Autodesk Inventor part; units mm, degrees
(part 3 of 5)
  line L1755 (-94.2698, 37.7318) -> (-93.9009, 37.14)
  line L1756 (-93.9009, 37.14) -> (-93.3437, 36.7396)
  line L1757 (-93.3437, 36.7396) -> (-92.5984, 36.5308)
  line L1758 (-92.5984, 36.5308) -> (-92.3338, 35.8693)
  line L1759 (-92.3338, 35.8693) -> (-93.5244, 33.2235)
  line L1760 (-93.5244, 33.2235) -> (-94.7873, 31.4902)
  line L1761 (-94.7873, 31.4902) -> (-95.5088, 29.5193)
  line L1762 (-95.5088, 29.5193) -> (-94.1859, 29.387)
  line L1763 (-94.1859, 29.387) -> (-93.4865, 28.8762)
  line L1764 (-93.4865, 28.8762) -> (-92.8566, 28.7721)
  line L1765 (-92.8566, 28.7721) -> (-92.2959, 29.0747)
  line L1766 (-92.2959, 29.0747) -> (-91.8046, 29.7839)
  line L1767 (-91.8046, 29.7839) -> (-92.3407, 30.6542)
  line L1768 (-92.3407, 30.6542) -> (-92.5855, 31.5617)
  line L1769 (-92.5855, 31.5617) -> (-92.5391, 32.5063)
  line L1770 (-92.5391, 32.5063) -> (-92.2015, 33.4881)
  line L1771 (-92.2015, 33.4881) -> (-91.5401, 33.7526)
  line L1772 (-91.5401, 33.7526) -> (-90.8786, 33.4881)
  line L1773 (-90.8786, 33.4881) -> (-90.2171, 30.0485)
  line L1774 (-90.2171, 30.0485) -> (-89.2902, 29.4549)
  line L1775 (-89.2902, 29.4549) -> (-88.6296, 28.5933)
  line L1776 (-88.6296, 28.5933) -> (-89.4059, 27.4096)
  line L1777 (-89.4059, 27.4096) -> (-90.3494, 26.3443)
  line L1778 (-90.3494, 26.3443) -> (-90.2708, 24.8832)
  line L1779 (-90.2708, 24.8832) -> (-90.399, 23.448)
  line L1780 (-90.399, 23.448) -> (-90.7339, 22.0389)
  line L1781 (-90.7339, 22.0389) -> (-91.2755, 20.6558)
  line L1782 (-91.2755, 20.6558) -> (-90.4507, 18.0829)
  line L1783 (-90.4507, 18.0829) -> (-89.1588, 15.761)
  line L1784 (-89.1588, 15.761) -> (-91.2755, 9.2787)
  line L1785 (-91.2755, 9.2787) -> (-91.0109, 8.6173)
  line L1786 (-91.0109, 8.6173) -> (-91.4592, 5.8191)
  line L1787 (-91.4592, 5.8191) -> (-92.0692, 3.061)
  line L1788 (-92.0692, 3.061) -> (-91.2286, 3.2382)
  line L1789 (-91.2286, 3.2382) -> (-90.614, 3.8548)
  line L1790 (-90.614, 3.8548) -> (-90.0294, 5.553)
  line L1791 (-90.0294, 5.553) -> (-89.0265, 7.0298)
  line L1792 (-89.0265, 7.0298) -> (-88.0062, 10.279)
  line L1793 (-88.0062, 10.279) -> (-87.439, 13.6444)
  line L1794 (-87.439, 13.6444) -> (-87.0421, 13.9089)
  line L1795 (-87.0421, 13.9089) -> (-86.9263, 10.5984)
  line L1796 (-86.9263, 10.5984) -> (-87.3067, 7.2944)
  line L1797 (-87.3067, 7.2944) -> (-87.1071, 5.8402)
  line L1798 (-87.1071, 5.8402) -> (-86.513, 4.5162)
  line L1799 (-86.513, 4.5162) -> (-87.5068, 1.3222)
  line L1800 (-87.5068, 1.3222) -> (-88.1005, -1.966)
  line L1801 (-29.0985, 51.4797) -> (-28.5184, 51.322)
  line L1802 (-28.5184, 51.322) -> (-28.0401, 50.9506)
  line L1803 (-28.0401, 50.9506) -> (-26.865, 49.3772)
  line L1804 (-26.865, 49.3772) -> (-25.9235, 47.6433)
  line L1805 (-25.9235, 47.6433) -> (-26.2095, 47.3714)
  line L1806 (-26.2095, 47.3714) -> (-26.5849, 47.2464)
  line L1807 (-26.5849, 47.2464) -> (-27.696, 47.8294)
  line L1808 (-27.696, 47.8294) -> (-28.7016, 48.5693)
  line L1809 (-28.7016, 48.5693) -> (-29.1503, 48.3856)
  line L1810 (-29.1503, 48.3856) -> (-29.4953, 48.0401)
  line L1811 (-29.4953, 48.0401) -> (-30.4738, 46.006)
  line L1812 (-30.4738, 46.006) -> (-31.612, 44.0714)
  line L1813 (-31.612, 44.0714) -> (-31.7443, 41.161)
  line L1814 (-31.7443, 41.161) -> (-32.8973, 41.4727)
  line L1815 (-32.8973, 41.4727) -> (-33.9933, 41.9547)
  line L1816 (-33.9933, 41.9547) -> (-34.3693, 45.4109)
  line L1817 (-34.3693, 45.4109) -> (-34.9193, 48.8339)
  line L1818 (-34.9193, 48.8339) -> (-34.6686, 49.4453)
  line L1819 (-34.6686, 49.4453) -> (-34.2984, 49.7814)
  line L1820 (-34.2984, 49.7814) -> (-33.8087, 49.8422)
  line L1821 (-33.8087, 49.8422) -> (-33.1995, 49.6276)
  line L1822 (-33.1995, 49.6276) -> (-32.2735, 45.9235)
  line L1823 (-32.2735, 45.9235) -> (-31.5452, 46.3563)
  line L1824 (-31.5452, 46.3563) -> (-31.1041, 46.9415)
  line L1825 (-31.1041, 46.9415) -> (-30.9499, 47.6792)
  line L1826 (-30.9499, 47.6792) -> (-31.0828, 48.5693)
  line L1827 (-31.0828, 48.5693) -> (-31.3153, 49.1092)
  line L1828 (-31.3153, 49.1092) -> (-31.3486, 49.6419)
  line L1829 (-31.3486, 49.6419) -> (-31.1829, 50.1675)
  line L1830 (-31.1829, 50.1675) -> (-30.8183, 50.686)
  line L1831 (-30.8183, 50.686) -> (-29.0985, 51.4797)
  line L1832 (-128.8463, 51.2151) -> (-125.6713, 51.2151)
  line L1833 (-125.6713, 51.2151) -> (-125.6713, 50.4214)
  line L1834 (-125.6713, 50.4214) -> (-128.5817, 50.2891)
  line L1835 (-128.5817, 50.2891) -> (-128.8138, 50.7213)
  line L1836 (-128.8138, 50.7213) -> (-128.8463, 51.2151)
  line L1837 (2.9161, 49.6276) -> (4.254, 49.6112)
  line L1838 (4.254, 49.6112) -> (5.5619, 49.3631)
  line L1839 (5.5619, 49.3631) -> (5.7224, 48.3373)
  line L1840 (5.7224, 48.3373) -> (5.6437, 47.356)
  line L1841 (5.6437, 47.356) -> (5.3256, 46.4191)
  line L1842 (5.3256, 46.4191) -> (4.7682, 45.5266)
  line L1843 (4.7682, 45.5266) -> (4.3713, 45.3942)
  line L1844 (4.3713, 45.3942) -> (3.9744, 45.5266)
  line L1845 (3.9744, 45.5266) -> (2.3869, 48.3047)
  line L1846 (2.3869, 48.3047) -> (2.9161, 49.6276)
  line L1847 (-138.1067, 49.3631) -> (-136.9146, 49.1321)
  line L1848 (-136.9146, 49.1321) -> (-135.8577, 48.5693)
  line L1849 (-135.8577, 48.5693) -> (-135.3932, 47.0503)
  line L1850 (-135.3932, 47.0503) -> (-135.3486, 45.5738)
  line L1851 (-135.3486, 45.5738) -> (-135.7239, 44.1398)
  line L1852 (-135.7239, 44.1398) -> (-136.5192, 42.7485)
  line L1853 (-136.5192, 42.7485) -> (-136.8754, 42.4036)
  line L1854 (-136.8754, 42.4036) -> (-137.2587, 42.2446)
  line L1855 (-137.2587, 42.2446) -> (-137.6691, 42.2714)
  line L1856 (-137.6691, 42.2714) -> (-138.1067, 42.4839)
  line L1857 (-138.1067, 42.4839) -> (-138.1067, 49.3631)
  line L1858 (-99.4775, 47.511) -> (-99.0469, 47.3511)
  line L1859 (-99.0469, 47.3511) -> (-99.213, 46.9818)
  line L1860 (-99.213, 46.9818) -> (-99.4374, 47.2048)
  line L1861 (-99.4374, 47.2048) -> (-99.4775, 47.511)
  line L1862 (-5.286, 47.511) -> (-4.2857, 47.4528)
  line L1863 (-4.2857, 47.4528) -> (-3.6656, 47.0806)
  line L1864 (-3.6656, 47.0806) -> (-3.4258, 46.3944)
  line L1865 (-3.4258, 46.3944) -> (-3.5662, 45.3943)
  line L1866 (-3.5662, 45.3943) -> (-4.0504, 45.0663)
  line L1867 (-4.0504, 45.0663) -> (-4.5205, 45.001)
  line L1868 (-4.5205, 45.001) -> (-4.9765, 45.1986)
  line L1869 (-4.9765, 45.1986) -> (-5.4183, 45.6589)
  line L1870 (-5.4183, 45.6589) -> (-5.5248, 46.6039)
  line L1871 (-5.5248, 46.6039) -> (-5.286, 47.511)
  line L1872 (-39.1526, -1.966) -> (-42.5922, -1.966)
  line L1873 (-42.5922, -1.966) -> (-43.411, -0.0639)
  line L1874 (-43.411, -0.0639) -> (-44.4443, 1.7381)
  line L1875 (-44.4443, 1.7381) -> (-45.0782, 0.9898)
  line L1876 (-45.0782, 0.9898) -> (-45.8187, 0.3876)
  line L1877 (-45.8187, 0.3876) -> (-46.6657, -0.0685)
  line L1878 (-46.6657, -0.0685) -> (-47.6193, -0.3785)
  line L1879 (-47.6193, -0.3785) -> (-47.8342, 0.5393)
  line L1880 (-47.8342, 0.5393) -> (-47.6193, 1.4735)
  line L1881 (-47.6193, 1.4735) -> (-48.2199, 3.2785)
  line L1882 (-48.2199, 3.2785) -> (-48.5745, 5.1149)
  line L1883 (-48.5745, 5.1149) -> (-48.683, 6.9827)
  line L1884 (-48.683, 6.9827) -> (-48.5453, 8.8819)
  line L1885 (-48.5453, 8.8819) -> (-47.487, 10.7339)
  line L1886 (-47.487, 10.7339) -> (-47.8531, 12.2631)
  line L1887 (-47.8531, 12.2631) -> (-48.6776, 13.6444)
  line L1888 (-48.6776, 13.6444) -> (-50.0005, 11.1308)
  line L1889 (-50.0005, 11.1308) -> (-50.5297, 10.9985)
  line L1890 (-50.5297, 10.9985) -> (-51.0589, 11.1308)
  line L1891 (-51.0589, 11.1308) -> (-51.8635, 11.9292)
  line L1892 (-51.8635, 11.9292) -> (-52.7786, 12.586)
  line L1893 (-52.7786, 12.586) -> (-53.0432, 14.4381)
  line L1894 (-53.0432, 14.4381) -> (-54.3038, 16.6946)
  line L1895 (-54.3038, 16.6946) -> (-55.2922, 19.0683)
  line L1896 (-55.2922, 19.0683) -> (-55.0552, 19.9474)
  line L1897 (-55.0552, 19.9474) -> (-55.4245, 20.7881)
  line L1898 (-55.4245, 20.7881) -> (-55.767, 21.0284)
  line L1899 (-55.767, 21.0284) -> (-56.0859, 20.7881)
  line L1900 (-56.0859, 20.7881) -> (-57.2766, 18.1423)
  line L1901 (-57.2766, 18.1423) -> (-57.8057, 17.8777)
  line L1902 (-57.8057, 17.8777) -> (-59.2517, 19.0586)
  line L1903 (-59.2517, 19.0586) -> (-60.5838, 20.3912)
  line L1904 (-60.5838, 20.3912) -> (-60.9904, 20.4558)
  line L1905 (-60.9904, 20.4558) -> (-61.3776, 20.2589)
  line L1906 (-61.3776, 20.2589) -> (-61.5149, 18.9486)
  line L1907 (-61.5149, 18.9486) -> (-61.3776, 17.6131)
  line L1908 (-61.3776, 17.6131) -> (-60.187, 16.8194)
  line L1909 (-60.187, 16.8194) -> (-59.7601, 14.1231)
  line L1910 (-59.7601, 14.1231) -> (-58.9963, 11.5277)
  line L1911 (-58.9963, 11.5277) -> (-59.4902, 11.4953)
  line L1912 (-59.4902, 11.4953) -> (-59.9224, 11.2631)
  line L1913 (-59.9224, 11.2631) -> (-60.2332, 10.2905)
  line L1914 (-60.2332, 10.2905) -> (-60.7778, 9.6135)
  line L1915 (-60.7778, 9.6135) -> (-61.5561, 9.2322)
  line L1916 (-61.5561, 9.2322) -> (-62.5682, 9.1464)
  line L1917 (-62.5682, 9.1464) -> (-62.7005, 8.2204)
  line L1918 (-62.7005, 8.2204) -> (-62.2318, 7.1909)
  line L1919 (-62.2318, 7.1909) -> (-61.9068, 6.1037)
  line L1920 (-61.9068, 6.1037) -> (-62.6567, 3.9438)
  line L1921 (-62.6567, 3.9438) -> (-63.2297, 1.7381)
  line L1922 (-63.2297, 1.7381) -> (-61.3776, 2.0027)
  line L1923 (-61.3776, 2.0027) -> (-61.3776, -1.966)
  line L1924 (-61.3776, -1.966) -> (-71.4317, -1.966)
  line L1925 (-71.4317, -1.966) -> (-71.564, -0.6431)
  line L1926 (-71.564, -0.6431) -> (-72.6447, 2.0679)
  line L1927 (-72.6447, 2.0679) -> (-73.1515, 4.9131)
  line L1928 (-73.1515, 4.9131) -> (-69.8443, 6.1037)
  line L1929 (-69.8443, 6.1037) -> (-68.9182, 7.0298)
  line L1930 (-68.9182, 7.0298) -> (-68.8851, 8.4843)
  line L1931 (-68.8851, 8.4843) -> (-68.4552, 9.6968)
  line L1932 (-68.4552, 9.6968) -> (-67.6284, 10.6671)
  line L1933 (-67.6284, 10.6671) -> (-66.4047, 11.3954)
  line L1934 (-66.4047, 11.3954) -> (-65.8755, 12.3214)
  line L1935 (-65.8755, 12.3214) -> (-66.2921, 13.0601)
  line L1936 (-66.2921, 13.0601) -> (-66.8278, 13.4606)
  line L1937 (-66.8278, 13.4606) -> (-67.4827, 13.5231)
  line L1938 (-67.4827, 13.5231) -> (-68.2568, 13.2475)
  line L1939 (-68.2568, 13.2475) -> (-69.0142, 11.6295)
  line L1940 (-69.0142, 11.6295) -> (-69.9943, 10.1862)
  line L1941 (-69.9943, 10.1862) -> (-71.197, 8.9175)
  line L1942 (-71.197, 8.9175) -> (-72.6224, 7.8235)
  line L1943 (-72.6224, 7.8235) -> (-73.0686, 8.8997)
  line L1944 (-73.0686, 8.8997) -> (-73.3496, 10.0081)
  line L1945 (-73.3496, 10.0081) -> (-73.4655, 11.1487)
  line L1946 (-73.4655, 11.1487) -> (-73.4161, 12.3214)
  line L1947 (-73.4161, 12.3214) -> (-72.1541, 12.3764)
  line L1948 (-72.1541, 12.3764) -> (-70.9026, 12.7183)
  line L1949 (-70.9026, 12.7183) -> (-70.0624, 13.4224)
  line L1950 (-70.0624, 13.4224) -> (-69.5398, 14.2524)
  line L1951 (-69.5398, 14.2524) -> (-69.3348, 15.2084)
  line L1952 (-69.3348, 15.2084) -> (-69.4474, 16.2902)
  line L1953 (-69.4474, 16.2902) -> (-70.7346, 17.8066)
  line L1954 (-70.7346, 17.8066) -> (-71.8286, 19.4652)
  line L1955 (-71.8286, 19.4652) -> (-71.9464, 20.3044)
  line L1956 (-71.9464, 20.3044) -> (-71.7652, 20.8487)
  line L1957 (-71.7652, 20.8487) -> (-71.2849, 21.0981)
  line L1958 (-71.2849, 21.0981) -> (-70.5057, 21.0527)
  line L1959 (-70.5057, 21.0527) -> (-69.8572, 18.8427)
  line L1960 (-69.8572, 18.8427) -> (-69.0505, 16.6871)
  line L1961 (-69.0505, 16.6871) -> (-68.6242, 16.5922)
  line L1962 (-68.6242, 16.5922) -> (-68.3057, 16.6708)
  line L1963 (-68.3057, 16.6708) -> (-68.0951, 16.9229)
  line L1964 (-68.0951, 16.9229) -> (-67.9922, 17.3485)
  line L1965 (-67.9922, 17.3485) -> (-69.1828, 21.0527)
  line L1966 (-69.1828, 21.0527) -> (-69.1924, 23.2536)
  line L1967 (-69.1924, 23.2536) -> (-69.4015, 23.9113)
  line L1968 (-69.4015, 23.9113) -> (-69.7468, 24.2739)
  line L1969 (-69.7468, 24.2739) -> (-70.2283, 24.3413)
  line L1970 (-70.2283, 24.3413) -> (-70.846, 24.1135)
  line L1971 (-70.846, 24.1135) -> (-72.4901, 22.7725)
  line L1972 (-72.4901, 22.7725) -> (-73.0881, 22.4538)
  line L1973 (-73.0881, 22.4538) -> (-73.5961, 22.4358)
  line L1974 (-73.5961, 22.4358) -> (-74.0142, 22.7184)
  line L1975 (-74.0142, 22.7184) -> (-74.3422, 23.3016)
  line L1976 (-74.3422, 23.3016) -> (-74.1545, 23.9851)
  line L1977 (-74.1545, 23.9851) -> (-74.136, 24.6539)
  line L1978 (-74.136, 24.6539) -> (-74.2868, 25.3081)
  line L1979 (-74.2868, 25.3081) -> (-74.6067, 25.9475)
  line L1980 (-74.6067, 25.9475) -> (-73.6247, 27.1948)
  line L1981 (-73.6247, 27.1948) -> (-72.4901, 28.3287)
  line L1982 (-72.4901, 28.3287) -> (-71.6214, 28.7579)
  line L1983 (-71.6214, 28.7579) -> (-70.979, 29.364)
  line L1984 (-70.979, 29.364) -> (-70.563, 30.1469)
  line L1985 (-70.563, 30.1469) -> (-70.3734, 31.1068)
  line L1986 (-70.3734, 31.1068) -> (-70.692, 31.5702)
  line L1987 (-70.692, 31.5702) -> (-70.8202, 32.0334)
  line L1988 (-70.8202, 32.0334) -> (-70.7581, 32.4963)
  line L1989 (-70.7581, 32.4963) -> (-70.5057, 32.9589)
  line L1990 (-70.5057, 32.9589) -> (-69.712, 29.7839)
  line L1991 (-69.712, 29.7839) -> (-68.0585, 28.7584)
  line L1992 (-68.0585, 28.7584) -> (-66.2724, 27.9318)
  line L1993 (-66.2724, 27.9318) -> (-65.8969, 28.0569)
  line L1994 (-65.8969, 28.0569) -> (-65.6109, 28.3287)
  line L1995 (-65.6109, 28.3287) -> (-66.4892, 30.4341)
  line L1996 (-66.4892, 30.4341) -> (-67.5953, 32.4297)
  line L1997 (-67.5953, 32.4297) -> (-67.7276, 35.2079)
  line L1998 (-67.7276, 35.2079) -> (-67.0661, 41.4256)
  line L1999 (-67.0661, 41.4256) -> (-64.9495, 44.0714)
  line L2000 (-64.9495, 44.0714) -> (-64.8172, 45.9235)
  line L2001 (-64.8172, 45.9235) -> (-64.0124, 45.8551)
  line L2002 (-64.0124, 45.8551) -> (-63.362, 45.3943)
  line L2003 (-63.362, 45.3943) -> (-63.0547, 44.8397)
  line L2004 (-63.0547, 44.8397) -> (-62.9744, 44.3021)
  line L2005 (-62.9744, 44.3021) -> (-63.1209, 43.7814)
  line L2006 (-63.1209, 43.7814) -> (-63.4943, 43.2777)
  line L2007 (-63.4943, 43.2777) -> (-63.2297, 43.0131)
  line L2008 (-63.2297, 43.0131) -> (-62.4004, 43.6928)
  line L2009 (-62.4004, 43.6928) -> (-61.3776, 44.0714)
  line L2010 (-61.3776, 44.0714) -> (-60.3274, 43.8086)
  line L2011 (-60.3274, 43.8086) -> (-59.4041, 43.9194)
  line L2012 (-59.4041, 43.9194) -> (-58.6076, 44.4039)
  line L2013 (-58.6076, 44.4039) -> (-57.938, 45.262)
  line L2014 (-57.938, 45.262) -> (-57.3205, 45.3719)
  line L2015 (-57.3205, 45.3719) -> (-56.7474, 45.1297)
  line L2016 (-56.7474, 45.1297) -> (-56.6151, 42.2193)
  line L2017 (-56.6151, 42.2193) -> (-56.9275, 41.0147)
  line L2018 (-56.9275, 41.0147) -> (-57.4726, 39.9737)
  line L2019 (-57.4726, 39.9737) -> (-58.2504, 39.0964)
  line L2020 (-58.2504, 39.0964) -> (-59.2609, 38.3829)
  line L2021 (-59.2609, 38.3829) -> (-64.1557, 36.1339)
  line L2022 (-64.1557, 36.1339) -> (-64.3891, 34.5696)
  line L2023 (-64.3891, 34.5696) -> (-64.1557, 32.9589)
  line L2024 (-64.1557, 32.9589) -> (-63.7676, 31.5253)
  line L2025 (-63.7676, 31.5253) -> (-62.9651, 30.3131)
  line L2026 (-62.9651, 30.3131) -> (-61.9068, 33.2235)
  line L2027 (-61.9068, 33.2235) -> (-61.5099, 32.9589)
  line L2028 (-61.5099, 32.9589) -> (-61.4954, 31.704)
  line L2029 (-61.4954, 31.704) -> (-61.6422, 30.4454)
  line L2030 (-61.6422, 30.4454) -> (-61.5301, 29.4351)
  line L2031 (-61.5301, 29.4351) -> (-61.2453, 28.461)
  line L2032 (-61.2453, 28.461) -> (-60.5728, 26.9609)
  line L2033 (-60.5728, 26.9609) -> (-59.6211, 25.7774)
  line L2034 (-59.6211, 25.7774) -> (-58.39, 24.9104)
  line L2035 (-58.39, 24.9104) -> (-56.8797, 24.36)
  line L2036 (-56.8797, 24.36) -> (-55.121, 23.3831)
  line L2037 (-55.121, 23.3831) -> (-53.4765, 22.2637)
  line L2038 (-53.4765, 22.2637) -> (-51.946, 21.0018)
  line L2039 (-51.946, 21.0018) -> (-50.5297, 19.5975)
  line L2040 (-50.5297, 19.5975) -> (-48.9521, 19.2457)
  line L2041 (-48.9521, 19.2457) -> (-47.3547, 19.4652)
  line L2042 (-47.3547, 19.4652) -> (-46.8255, 20.7881)
  line L2043 (-46.8255, 20.7881) -> (-48.1484, 22.5079)
  line L2044 (-48.1484, 22.5079) -> (-47.7516, 22.9048)
  line L2045 (-47.7516, 22.9048) -> (-46.2964, 21.8464)
  line L2046 (-46.2964, 21.8464) -> (-45.9219, 22.0886)
  line L2047 (-45.9219, 22.0886) -> (-45.7672, 22.5079)
  line L2048 (-45.7672, 22.5079) -> (-46.8255, 25.5506)
  line L2049 (-46.8255, 25.5506) -> (-46.2964, 26.3443)
  line L2050 (-46.2964, 26.3443) -> (-45.8113, 25.9916)
  line L2051 (-45.8113, 25.9916) -> (-45.238, 25.8152)
  line L2052 (-45.238, 25.8152) -> (-43.8134, 26.5477)
  line L2053 (-43.8134, 26.5477) -> (-43.391, 26.9954)
  line L2054 (-43.391, 26.9954) -> (-43.162, 27.4974)
  line L2055 (-43.162, 27.4974) -> (-43.1264, 28.0537)
  line L2056 (-43.1264, 28.0537) -> (-43.2841, 28.6643)
  line L2057 (-43.2841, 28.6643) -> (-44.1797, 30.0485)
  line L2058 (-44.1797, 30.0485) -> (-43.5366, 30.306)
  line L2059 (-43.5366, 30.306) -> (-42.8568, 30.1808)
  line L2060 (-42.8568, 30.1808) -> (-41.9146, 29.5033)
  line L2061 (-41.9146, 29.5033) -> (-40.8724, 28.9902)
  line L2062 (-40.8724, 28.9902) -> (-40.3009, 29.6426)
  line L2063 (-40.3009, 29.6426) -> (-39.9464, 30.4454)
  line L2064 (-39.9464, 30.4454) -> (-39.1491, 30.1661)
  line L2065 (-39.1491, 30.1661) -> (-38.729, 29.6982)
  line L2066 (-38.729, 29.6982) -> (-38.6861, 29.0417)
  line L2067 (-38.6861, 29.0417) -> (-39.0203, 28.1964)
  line L2068 (-39.0203, 28.1964) -> (-40.3059, 27.1131)
  line L2069 (-40.3059, 27.1131) -> (-41.1816, 26.0747)
  line L2070 (-41.1816, 26.0747) -> (-41.6475, 25.0813)
  line L2071 (-41.6475, 25.0813) -> (-41.7036, 24.1328)
  line L2072 (-41.7036, 24.1328) -> (-41.3499, 23.2292)
  line L2073 (-41.3499, 23.2292) -> (-40.5863, 22.3706)
  line L2074 (-40.5863, 22.3706) -> (-39.4129, 21.5569)
  line L2075 (-39.4129, 21.5569) -> (-37.8297, 20.7881)
  line L2076 (-37.8297, 20.7881) -> (-37.5934, 19.1841)
  line L2077 (-37.5934, 19.1841) -> (-37.962, 17.6131)
  line L2078 (-37.962, 17.6131) -> (-38.9851, 16.5591)
  line L2079 (-38.9851, 16.5591) -> (-39.7451, 15.3698)
  line L2080 (-39.7451, 15.3698) -> (-40.2419, 14.0455)
  line L2081 (-40.2419, 14.0455) -> (-40.4755, 12.586)
  line L2082 (-40.4755, 12.586) -> (-39.4851, 12.7013)
  line L2083 (-39.4851, 12.7013) -> (-38.7557, 13.3798)
  line L2084 (-38.7557, 13.3798) -> (-38.0966, 13.1876)
  line L2085 (-38.0966, 13.1876) -> (-37.48, 13.2118)
  line L2086 (-37.48, 13.2118) -> (-36.906, 13.4522)
  line L2087 (-36.906, 13.4522) -> (-36.3745, 13.9089)
  line L2088 (-36.3745, 13.9089) -> (-36.5397, 14.623)
  line L2089 (-36.5397, 14.623) -> (-36.8815, 15.2137)
  line L2090 (-36.8815, 15.2137) -> (-37.3997, 15.6813)
  line L2091 (-37.3997, 15.6813) -> (-38.0943, 16.0256)
  line L2092 (-38.0943, 16.0256) -> (-36.9086, 16.0817)
  line L2093 (-36.9086, 16.0817) -> (-35.713, 15.761)
  line L2094 (-35.713, 15.761) -> (-34.1364, 13.789)
  line L2095 (-34.1364, 13.789) -> (-32.8026, 11.66)
  line L2096 (-32.8026, 11.66) -> (-33.0886, 11.3881)
  line L2097 (-33.0886, 11.3881) -> (-33.4641, 11.2631)
  line L2098 (-33.4641, 11.2631) -> (-34.2564, 12.3146)
  line L2099 (-34.2564, 12.3146) -> (-35.3162, 13.1152)
  line L2100 (-35.3162, 13.1152) -> (-37.0454, 11.9188)
  line L2101 (-37.0454, 11.9188) -> (-38.888, 10.8662)
  line L2102 (-38.888, 10.8662) -> (-39.4254, 10.189)
  line L2103 (-39.4254, 10.189) -> (-39.8141, 9.411)
  line L2104 (-39.8141, 9.411) -> (-39.9464, 7.8235)
  line L2105 (-39.9464, 7.8235) -> (-39.8141, 6.236)
  line L2106 (-39.8141, 6.236) -> (-39.1334, 4.1972)
  line L2107 (-39.1334, 4.1972) -> (-38.7963, 2.1506)
  line L2108 (-38.7963, 2.1506) -> (-38.8027, 0.0962)
  line L2109 (-38.8027, 0.0962) -> (-39.1526, -1.966)
  line L2110 (-60.8484, 41.9547) -> (-60.4908, 41.6278)
  line L2111 (-60.4908, 41.6278) -> (-60.3496, 41.2543)
  line L2112 (-60.3496, 41.2543) -> (-60.4247, 40.8341)
  line L2113 (-60.4247, 40.8341) -> (-60.7161, 40.3672)
  line L2114 (-60.7161, 40.3672) -> (-61.4786, 39.6471)
  line L2115 (-61.4786, 39.6471) -> (-62.328, 39.0983)
  line L2116 (-62.328, 39.0983) -> (-63.2645, 38.721)
  line L2117 (-63.2645, 38.721) -> (-64.288, 38.5152)
  line L2118 (-64.288, 38.5152) -> (-64.1557, 39.3089)
  line L2119 (-64.1557, 39.3089) -> (-62.5426, 40.7071)
  line L2120 (-62.5426, 40.7071) -> (-60.8484, 41.9547)
  line L2121 (-100.0067, 41.6902) -> (-100.0783, 40.9799)
  line L2122 (-100.0783, 40.9799) -> (-100.3006, 40.3022)
  line L2123 (-100.3006, 40.3022) -> (-101.1973, 39.0443)
  line L2124 (-101.1973, 39.0443) -> (-101.1956, 39.8486)
  line L2125 (-101.1956, 39.8486) -> (-100.9328, 40.6318)
  line L2126 (-100.9328, 40.6318) -> (-100.0067, 41.6902)
  line L2127 (-104.5046, 39.8381) -> (-103.1817, 39.8381)
  line L2128 (-103.1817, 39.8381) -> (-103.709, 37.9901)
  line L2129 (-103.709, 37.9901) -> (-104.7692, 36.3985)
  line L2130 (-104.7692, 36.3985) -> (-105.1974, 36.8313)
  line L2131 (-105.1974, 36.8313) -> (-105.2984, 37.4568)
  line L2132 (-105.2984, 37.4568) -> (-105.0188, 38.6925)
  line L2133 (-105.0188, 38.6925) -> (-104.5046, 39.8381)
  line L2134 (-138.1067, 37.1922) -> (-138.1067, 38.5152)
  line L2135 (-138.1067, 38.5152) -> (-136.916, 39.0443)
  line L2136 (-136.916, 39.0443) -> (-136.7165, 38.3251)
  line L2137 (-136.7165, 38.3251) -> (-136.8484, 37.7767)
  line L2138 (-136.8484, 37.7767) -> (-137.3118, 37.3991)
  line L2139 (-137.3118, 37.3991) -> (-138.1067, 37.1922)
  line L2140 (-39.6818, 38.7797) -> (-39.1108, 38.5226)
  line L2141 (-39.1108, 38.5226) -> (-38.6559, 38.1502)
  line L2142 (-38.6559, 38.1502) -> (-38.317, 37.6627)
  line L2143 (-38.317, 37.6627) -> (-38.0943, 37.06)
  line L2144 (-38.0943, 37.06) -> (-38.5656, 34.6375)
  line L2145 (-38.5656, 34.6375) -> (-38.6235, 32.1652)
  line L2146 (-38.6235, 32.1652) -> (-39.4172, 32.1652)
  line L2147 (-39.4172, 32.1652) -> (-39.4847, 34.9635)
  line L2148 (-39.4847, 34.9635) -> (-39.9464, 37.7214)
  line L2149 (-39.9464, 37.7214) -> (-39.6818, 38.7797)
  line L2150 (-88.6296, 38.5152) -> (-88.2776, 38.1711)
  line L2151 (-88.2776, 38.1711) -> (-88.1381, 37.7919)
  line L2152 (-88.1381, 37.7919) -> (-88.2114, 37.3774)
  line L2153 (-88.2114, 37.3774) -> (-88.4974, 36.9277)
  line L2154 (-88.4974, 36.9277) -> (-88.7735, 37.3044)
  line L2155 (-88.7735, 37.3044) -> (-88.8875, 37.6946)
  line L2156 (-88.8875, 37.6946) -> (-88.8396, 38.0982)
  line L2157 (-88.8396, 38.0982) -> (-88.6296, 38.5152)
  line L2158 (-30.686, 38.2506) -> (-29.9159, 38.1267)
  line L2159 (-29.9159, 38.1267) -> (-29.3631, 37.5891)
  line L2160 (-29.3631, 37.5891) -> (-30.2158, 36.8972)
  line L2161 (-30.2158, 36.8972) -> (-31.2151, 36.3985)
  line L2162 (-31.2151, 36.3985) -> (-31.6918, 36.6364)
  line L2163 (-31.6918, 36.6364) -> (-32.0089, 37.06)
  line L2164 (-32.0089, 37.06) -> (-31.4936, 37.8408)
  line L2165 (-31.4936, 37.8408) -> (-30.686, 38.2506)
  line L2166 (-75.9297, 37.986) -> (-75.4833, 37.7651)
  line L2167 (-75.4833, 37.7651) -> (-75.2905, 37.5151)
  line L2168 (-75.2905, 37.5151) -> (-75.3511, 37.2359)
  line L2169 (-75.3511, 37.2359) -> (-75.6651, 36.9277)
  line L2170 (-75.6651, 36.9277) -> (-76.0638, 37.4359)
  line L2171 (-76.0638, 37.4359) -> (-75.9297, 37.986)
  line L2172 (-36.2422, 36.6631) -> (-35.2269, 34.9039)
  line L2173 (-35.2269, 34.9039) -> (-33.9933, 33.2235)
  line L2174 (-33.9933, 33.2235) -> (-33.7371, 31.941)
  line L2175 (-33.7371, 31.941) -> (-33.3318, 30.71)
  line L2176 (-33.3318, 30.71) -> (-33.5964, 30.5777)
  line L2177 (-33.5964, 30.5777) -> (-36.3745, 35.6047)
  line L2178 (-36.3745, 35.6047) -> (-36.4563, 36.1528)
  line L2179 (-36.4563, 36.1528) -> (-36.2422, 36.6631)
  line L2180 (-88.8942, 35.8693) -> (-88.6606, 35.2042)
  line L2181 (-88.6606, 35.2042) -> (-89.0265, 34.5464)
  line L2182 (-89.0265, 34.5464) -> (-89.0697, 35.2138)
  line L2183 (-89.0697, 35.2138) -> (-88.8942, 35.8693)
  line L2184 (-138.1067, 35.0756) -> (-137.5271, 34.9738)
  line L2185 (-137.5271, 34.9738) -> (-137.1575, 34.6973)
  line L2186 (-137.1575, 34.6973) -> (-136.998, 34.2462)
  line L2187 (-136.998, 34.2462) -> (-137.0483, 33.6204)
  line L2188 (-137.0483, 33.6204) -> (-137.4797, 31.5928)
  line L2189 (-137.4797, 31.5928) -> (-137.7098, 29.5193)
  line L2190 (-137.7098, 29.5193) -> (-138.1067, 28.9902)
  line L2191 (-138.1067, 28.9902) -> (-138.1067, 35.0756)
  line L2192 (-46.5609, 33.7527) -> (-46.198, 33.7035)
  line L2193 (-46.198, 33.7035) -> (-45.8995, 33.4881)
  line L2194 (-45.8995, 33.4881) -> (-45.3468, 32.5016)
  line L2195 (-45.3468, 32.5016) -> (-45.2508, 31.5994)
  line L2196 (-45.2508, 31.5994) -> (-45.6114, 30.7817)
  line L2197 (-45.6114, 30.7817) -> (-46.4287, 30.0485)
  line L2198 (-46.4287, 30.0485) -> (-46.6932, 28.1964)
  line L2199 (-46.6932, 28.1964) -> (-47.1908, 29.5963)
  line L2200 (-47.1908, 29.5963) -> (-47.3346, 30.989)
  line L2201 (-47.3346, 30.989) -> (-47.1247, 32.3745)
  line L2202 (-47.1247, 32.3745) -> (-46.5609, 33.7527)
  line L2203 (-31.7443, 32.6943) -> (-31.1432, 32.3592)
  line L2204 (-31.1432, 32.3592) -> (-30.7224, 31.8947)
  line L2205 (-30.7224, 31.8947) -> (-30.4818, 31.3008)
  line L2206 (-30.4818, 31.3008) -> (-30.4214, 30.5777)
  line L2207 (-30.4214, 30.5777) -> (-31.2528, 30.8111)
  line L2208 (-31.2528, 30.8111) -> (-31.7505, 31.2417)
  line L2209 (-31.7505, 31.2417) -> (-31.9143, 31.8694)
  line L2210 (-31.9143, 31.8694) -> (-31.7443, 32.6943)
  line L2211 (-76.7234, 32.4297) -> (-76.3766, 32.0976)
  line L2212 (-76.3766, 32.0976) -> (-76.217, 31.7223)
  line L2213 (-76.217, 31.7223) -> (-76.2444, 31.3039)
  line L2214 (-76.2444, 31.3039) -> (-76.4588, 30.8423)
  line L2215 (-76.4588, 30.8423) -> (-77.1877, 30.3952)
  line L2216 (-77.1877, 30.3952) -> (-78.0463, 30.3131)
  line L2217 (-78.0463, 30.3131) -> (-77.914, 31.1068)
  line L2218 (-77.914, 31.1068) -> (-76.7234, 32.4297)
  line L2219 (-78.3109, 29.7839) -> (-77.9845, 29.5899)
  line L2220 (-77.9845, 29.5899) -> (-77.7817, 29.2548)
  line L2221 (-77.7817, 29.2548) -> (-78.0701, 28.5142)
  line L2222 (-78.0701, 28.5142) -> (-78.5755, 27.9318)
  line L2223 (-78.5755, 27.9318) -> (-78.7593, 28.4345)
  line L2224 (-78.7593, 28.4345) -> (-78.7764, 28.9108)
  line L2225 (-78.7764, 28.9108) -> (-78.6269, 29.3605)
  line L2226 (-78.6269, 29.3605) -> (-78.3109, 29.7839)
  line L2227 (-55.5568, 29.7839) -> (-54.55, 29.7043)
  line L2228 (-54.55, 29.7043) -> (-53.9057, 29.325)
  line L2229 (-53.9057, 29.325) -> (-53.624, 28.6459)
  line L2230 (-53.624, 28.6459) -> (-53.7047, 27.6673)
  line L2231 (-53.7047, 27.6673) -> (-52.9109, 25.6829)
  line L2232 (-52.9109, 25.6829) -> (-53.3004, 25.0688)
  line L2233 (-53.3004, 25.0688) -> (-53.7829, 24.7759)
  line L2234 (-53.7829, 24.7759) -> (-54.3587, 24.8042)
  line L2235 (-54.3587, 24.8042) -> (-55.0276, 25.1537)
  line L2236 (-55.0276, 25.1537) -> (-56.1285, 25.969)
  line L2237 (-56.1285, 25.969) -> (-57.4088, 26.4766)
  line L2238 (-57.4088, 26.4766) -> (-58.1365, 27.0719)
  line L2239 (-58.1365, 27.0719) -> (-58.7318, 27.7995)
  line L2240 (-58.7318, 27.7995) -> (-55.5568, 29.7839)
  line L2241 (-48.9422, 29.2548) -> (-48.3947, 29.2195)
  line L2242 (-48.3947, 29.2195) -> (-48.0358, 29.0093)
  line L2243 (-48.0358, 29.0093) -> (-47.8655, 28.6242)
  line L2244 (-47.8655, 28.6242) -> (-47.8839, 28.0641)
  line L2245 (-47.8839, 28.0641) -> (-48.0912, 27.3259)
  line L2246 (-48.0912, 27.3259) -> (-48.6776, 26.8735)
  line L2247 (-48.6776, 26.8735) -> (-49.1058, 27.3063)
  line L2248 (-49.1058, 27.3063) -> (-49.2068, 27.9318)
  line L2249 (-49.2068, 27.9318) -> (-48.9422, 29.2548)
  line L2250 (3.4452, 28.1964) -> (3.8214, 27.9279)
  line L2251 (3.8214, 27.9279) -> (3.9689, 27.6179)
  line L2252 (3.9689, 27.6179) -> (3.8876, 27.2665)
  line L2253 (3.8876, 27.2665) -> (3.5775, 26.8735)
  line L2254 (3.5775, 26.8735) -> (3.1807, 27.535)
  line L2255 (3.1807, 27.535) -> (3.3961, 27.8334)
  line L2256 (3.3961, 27.8334) -> (3.4452, 28.1964)
  line L2257 (-136.5192, 27.9318) -> (-136.069, 27.6951)
  line L2258 (-136.069, 27.6951) -> (-135.8528, 27.3957)
  line L2259 (-135.8528, 27.3957) -> (-135.8705, 27.0336)
  line L2260 (-135.8705, 27.0336) -> (-136.1223, 26.6089)
  line L2261 (-136.1223, 26.6089) -> (-136.4734, 27.2184)
  line L2262 (-136.4734, 27.2184) -> (-136.5192, 27.9318)
  line L2263 (-33.0672, 27.6673) -> (-32.3945, 27.5753)
  line L2264 (-32.3945, 27.5753) -> (-31.8766, 27.1381)
  line L2265 (-31.8766, 27.1381) -> (-31.5289, 26.1101)
  line L2266 (-31.5289, 26.1101) -> (-31.4797, 25.0214)
  line L2267 (-31.4797, 25.0214) -> (-32.2327, 25.158)
  line L2268 (-32.2327, 25.158) -> (-32.7924, 25.5122)
  line L2269 (-32.7924, 25.5122) -> (-33.1588, 26.084)
  line L2270 (-33.1588, 26.084) -> (-33.3318, 26.8735)
  line L2271 (-33.3318, 26.8735) -> (-33.0672, 27.6673)
  line L2272 (15.3515, 25.5506) -> (16.1452, 25.5506)
  line L2273 (16.1452, 25.5506) -> (16.0959, 24.7308)
  line L2274 (16.0959, 24.7308) -> (15.9031, 24.3693)
  line L2275 (15.9031, 24.3693) -> (15.5668, 24.4662)
  line L2276 (15.5668, 24.4662) -> (15.0869, 25.0214)
  line L2277 (15.0869, 25.0214) -> (15.3515, 25.5506)
  line L2278 (-106.6213, 25.286) -> (-106.0921, 24.6245)
  line L2279 (-106.0921, 24.6245) -> (-106.5342, 24.7526)
  line L2280 (-106.5342, 24.7526) -> (-106.6213, 25.286)
  line L2281 (-22.7485, 25.286) -> (-21.161, 25.1537)
  line L2282 (-21.161, 25.1537) -> (-18.795, 23.7064)
  line L2283 (-18.795, 23.7064) -> (-16.5308, 22.111)
  line L2284 (-16.5308, 22.111) -> (-15.7187, 22.1345)
  line L2285 (-15.7187, 22.1345) -> (-15.007, 21.9218)
  line L2286 (-15.007, 21.9218) -> (-14.3958, 21.4731)
  line L2287 (-14.3958, 21.4731) -> (-13.8849, 20.7881)
  line L2288 (-13.8849, 20.7881) -> (-13.7631, 20.237)
  line L2289 (-13.7631, 20.237) -> (-14.0172, 19.7298)
  line L2290 (-14.0172, 19.7298) -> (-16.5308, 21.8464)
  line L2291 (-16.5308, 21.8464) -> (-17.4638, 21.7047)
  line L2292 (-17.4638, 21.7047) -> (-18.3701, 21.7677)
  line L2293 (-18.3701, 21.7677) -> (-19.2497, 22.0354)
  line L2294 (-19.2497, 22.0354) -> (-20.1026, 22.5079)
  line L2295 (-20.1026, 22.5079) -> (-21.2859, 23.6052)
  line L2296 (-21.2859, 23.6052) -> (-22.6162, 24.4923)
  line L2297 (-22.6162, 24.4923) -> (-22.7485, 25.286)
  line L2298 (-134.1379, 24.4923) -> (-133.7072, 24.3324)
  line L2299 (-133.7072, 24.3324) -> (-133.8733, 23.9631)
  line L2300 (-133.8733, 23.9631) -> (-134.0977, 24.1861)
  line L2301 (-134.0977, 24.1861) -> (-134.1379, 24.4923)
  line L2302 (-62.9651, 24.4923) -> (-61.7836, 23.9769)
  line L2303 (-61.7836, 23.9769) -> (-60.8484, 23.0371)
  line L2304 (-60.8484, 23.0371) -> (-59.9471, 23.0571)
  line L2305 (-59.9471, 23.0571) -> (-59.2718, 22.7771)
  line L2306 (-59.2718, 22.7771) -> (-58.8226, 22.1972)
  line L2307 (-58.8226, 22.1972) -> (-58.5995, 21.3173)
  line L2308 (-58.5995, 21.3173) -> (-60.3193, 20.7881)
  line L2309 (-60.3193, 20.7881) -> (-62.7005, 21.7141)
  line L2310 (-62.7005, 21.7141) -> (-63.0381, 22.3746)
  line L2311 (-63.0381, 22.3746) -> (-63.1947, 23.0578)
  line L2312 (-63.1947, 23.0578) -> (-63.1703, 23.7636)
  line L2313 (-63.1703, 23.7636) -> (-62.9651, 24.4923)
  line L2314 (-1.0527, 24.4923) -> (-0.6763, 24.3761)
  line L2315 (-0.6763, 24.3761) -> (-0.5288, 24.2051)
  line L2316 (-0.5288, 24.2051) -> (-0.9204, 23.6985)
  line L2317 (-0.9204, 23.6985) -> (-1.0527, 24.4923)
  line L2318 (-124.3483, 23.9631) -> (-123.5943, 24.0318)
  line L2319 (-123.5943, 24.0318) -> (-123.0343, 23.8341)
  line L2320 (-123.0343, 23.8341) -> (-122.6683, 23.3703)
  line L2321 (-122.6683, 23.3703) -> (-122.4963, 22.6402)
  line L2322 (-122.4963, 22.6402) -> (-123.1544, 21.5826)
  line L2323 (-123.1544, 21.5826) -> (-123.5546, 20.3912)
  line L2324 (-123.5546, 20.3912) -> (-125.6713, 19.7298)
  line L2325 (-125.6713, 19.7298) -> (-126.7854, 20.4467)
  line L2326 (-126.7854, 20.4467) -> (-127.7879, 21.3173)
  line L2327 (-127.7879, 21.3173) -> (-127.1265, 21.5818)
  line L2328 (-127.1265, 21.5818) -> (-124.6129, 21.0527)
  line L2329 (-124.6129, 21.0527) -> (-124.7407, 21.8332)
  line L2330 (-124.7407, 21.8332) -> (-125.1421, 22.5079)
  line L2331 (-125.1421, 22.5079) -> (-124.8198, 23.2854)
  line L2332 (-124.8198, 23.2854) -> (-124.3483, 23.9631)
  line L2333 (-11.1068, 23.6985) -> (-10.2477, 23.4032)
  line L2334 (-10.2477, 23.4032) -> (-9.8732, 22.9961)
  line L2335 (-9.8732, 22.9961) -> (-9.9831, 22.4772)
  line L2336 (-9.9831, 22.4772) -> (-10.5777, 21.8464)
  line L2337 (-10.5777, 21.8464) -> (-11.2099, 22.2087)
  line L2338 (-11.2099, 22.2087) -> (-11.5089, 22.6381)
  line L2339 (-11.5089, 22.6381) -> (-11.4745, 23.1348)
  line L2340 (-11.4745, 23.1348) -> (-11.1068, 23.6985)
  line L2341 (-89.688, 22.9048) -> (-89.1941, 22.8724)
  line L2342 (-89.1941, 22.8724) -> (-88.7619, 22.6402)
  line L2343 (-88.7619, 22.6402) -> (-87.5713, 20.5235)
  line L2344 (-87.5713, 20.5235) -> (-87.9031, 20.1759)
  line L2345 (-87.9031, 20.1759) -> (-88.2563, 20.06)
  line L2346 (-88.2563, 20.06) -> (-88.6307, 20.1759)
  line L2347 (-88.6307, 20.1759) -> (-89.0265, 20.5235)
  line L2348 (-89.0265, 20.5235) -> (-89.5705, 21.6558)
  line L2349 (-89.5705, 21.6558) -> (-89.688, 22.9048)
  line L2350 (-5.8152, -1.966) -> (-14.2818, -1.966)
  line L2351 (-14.2818, -1.966) -> (-14.1743, -0.2873)
  line L2352 (-14.1743, -0.2873) -> (-13.7527, 1.3412)
  line L2353 (-13.7527, 1.3412) -> (-13.8627, 1.9026)
  line L2354 (-13.8627, 1.9026) -> (-14.2818, 2.2673)
  line L2355 (-14.2818, 2.2673) -> (-15.737, 0.4152)
  line L2356 (-15.737, 0.4152) -> (-15.8693, -1.966)
  line L2357 (-15.8693, -1.966) -> (-24.8651, -1.966)
  line L2358 (-24.8651, -1.966) -> (-25.4768, -0.9551)
  line L2359 (-25.4768, -0.9551) -> (-25.9235, 0.1506)
  line L2360 (-25.9235, 0.1506) -> (-25.1762, 1.909)
  line L2361 (-25.1762, 1.909) -> (-24.6006, 3.7225)
  line L2362 (-24.6006, 3.7225) -> (-24.7328, 4.6485)
  line L2363 (-24.7328, 4.6485) -> (-25.262, 5.0454)
  line L2364 (-25.262, 5.0454) -> (-25.6589, 5.5746)
  line L2365 (-25.6589, 5.5746) -> (-25.5558, 6.4664)
  line L2366 (-25.5558, 6.4664) -> (-25.3009, 7.2928)
  line L2367 (-25.3009, 7.2928) -> (-24.8943, 8.0539)
  line L2368 (-24.8943, 8.0539) -> (-24.336, 8.7496)
  line L2369 (-24.336, 8.7496) -> (-23.1911, 9.3675)
  line L2370 (-23.1911, 9.3675) -> (-22.2193, 10.2048)
  line L2371 (-22.2193, 10.2048) -> (-22.4839, 10.6017)
  line L2372 (-22.4839, 10.6017) -> (-25.1297, 11.3954)
  line L2373 (-25.1297, 11.3954) -> (-25.5266, 12.0569)
  line L2374 (-25.5266, 12.0569) -> (-25.8733, 14.9576)
  line L2375 (-25.8733, 14.9576) -> (-25.7912, 17.8777)
  line L2376 (-25.7912, 17.8777) -> (-25.1274, 18.1853)
  line L2377 (-25.1274, 18.1853) -> (-24.6006, 18.6714)
  line L2378 (-24.6006, 18.6714) -> (-25.2294, 19.4798)
  line L2379 (-25.2294, 19.4798) -> (-25.5933, 20.3666)
  line L2380 (-25.5933, 20.3666) -> (-25.6924, 21.3319)
  line L2381 (-25.6924, 21.3319) -> (-25.5266, 22.3756)
  line L2382 (-25.5266, 22.3756) -> (-25.1297, 22.6402)
  line L2383 (-25.1297, 22.6402) -> (-24.1862, 22.076)
  line L2384 (-24.1862, 22.076) -> (-23.5422, 21.185)
  line L2385 (-23.5422, 21.185) -> (-21.9547, 20.9204)
  line L2386 (-21.9547, 20.9204) -> (-21.5088, 20.574)
  line L2387 (-21.5088, 20.574) -> (-21.272, 20.1719)
  line L2388 (-21.272, 20.1719) -> (-21.2443, 19.7141)
  line L2389 (-21.2443, 19.7141) -> (-21.4256, 19.2006)
  line L2390 (-21.4256, 19.2006) -> (-22.1661, 18.9123)
  line L2391 (-22.1661, 18.9123) -> (-22.7485, 18.4068)
  line L2392 (-22.7485, 18.4068) -> (-21.5972, 16.8588)
  line L2393 (-21.5972, 16.8588) -> (-20.2349, 15.4964)
  line L2394 (-20.2349, 15.4964) -> (-18.6474, 18.4068)
  line L2395 (-18.6474, 18.4068) -> (-18.2506, 18.6714)
  line L2396 (-18.2506, 18.6714) -> (-17.8537, 18.4068)
  line L2397 (-17.8537, 18.4068) -> (-17.5891, 16.2902)
  line L2398 (-17.5891, 16.2902) -> (-14.9433, 10.4694)
  line L2399 (-14.9433, 10.4694) -> (-13.4881, 9.0142)
  line L2400 (-13.4881, 9.0142) -> (-12.6256, 8.9641)
  line L2401 (-12.6256, 8.9641) -> (-11.7683, 9.1464)
  line L2402 (-11.7683, 9.1464) -> (-11.1642, 9.0262)
  line L2403 (-11.1642, 9.0262) -> (-10.7099, 8.6173)
  line L2404 (-10.7099, 8.6173) -> (-11.0517, 5.8671)
  line L2405 (-11.0517, 5.8671) -> (-10.9745, 3.061)
  line L2406 (-10.9745, 3.061) -> (-10.7265, 1.82)
  line L2407 (-10.7265, 1.82) -> (-10.1808, 0.6798)
  line L2408 (-10.1808, 0.6798) -> (-9.8195, -0.0145)
  line L2409 (-9.8195, -0.0145) -> (-9.3243, -0.4444)
  line L2410 (-9.3243, -0.4444) -> (-8.6951, -0.6098)
  line L2411 (-8.6951, -0.6098) -> (-7.9318, -0.5108)
  line L2412 (-7.9318, -0.5108) -> (-6.6089, 2.0027)
  line L2413 (-6.6089, 2.0027) -> (-5.9384, 0.086)
  line L2414 (-5.9384, 0.086) -> (-5.8152, -1.966)
  line L2415 (1.3286, 22.6402) -> (2.3869, 22.6402)
  line L2416 (2.3869, 22.6402) -> (2.456, 21.8498)
  line L2417 (2.456, 21.8498) -> (2.2805, 21.1894)
  line L2418 (2.2805, 21.1894) -> (1.8607, 20.6591)
  line L2419 (1.8607, 20.6591) -> (1.1963, 20.2589)
  line L2420 (1.1963, 20.2589) -> (1.0833, 21.4678)
  line L2421 (1.0833, 21.4678) -> (1.3286, 22.6402)
  line L2422 (-138.1067, 21.8464) -> (-137.3657, 21.8515)
  line L2423 (-137.3657, 21.8515) -> (-136.7219, 21.6547)
  line L2424 (-136.7219, 21.6547) -> (-136.1751, 21.2562)
  line L2425 (-136.1751, 21.2562) -> (-135.7254, 20.6558)
  line L2426 (-135.7254, 20.6558) -> (-135.2614, 20.6188)
  line L2427 (-135.2614, 20.6188) -> (-134.7994, 20.7881)
  line L2428 (-134.7994, 20.7881) -> (-134.2737, 20.5353)
  line L2429 (-134.2737, 20.5353) -> (-133.9882, 20.1864)
  line L2430 (-133.9882, 20.1864) -> (-133.9429, 19.7415)
  line L2431 (-133.9429, 19.7415) -> (-134.1379, 19.2006)
  line L2432 (-134.1379, 19.2006) -> (-134.8785, 18.9123)
  line L2433 (-134.8785, 18.9123) -> (-135.4608, 18.4068)
  line L2434 (-135.4608, 18.4068) -> (-134.0308, 16.6044)
  line L2435 (-134.0308, 16.6044) -> (-132.4181, 14.9673)
  line L2436 (-132.4181, 14.9673) -> (-132.3921, 12.5803)
  line L2437 (-132.3921, 12.5803) -> (-132.6827, 10.2048)
  line L2438 (-132.6827, 10.2048) -> (-133.2475, 9.8893)
  line L2439 (-133.2475, 9.8893) -> (-133.6783, 9.4754)
  line L2440 (-133.6783, 9.4754) -> (-133.9751, 8.9632)
  line L2441 (-133.9751, 8.9632) -> (-134.1379, 8.3527)
  line L2442 (-134.1379, 8.3527) -> (-132.5504, 5.5746)
  line L2443 (-132.5504, 5.5746) -> (-131.8823, 5.5327)
  line L2444 (-131.8823, 5.5327) -> (-131.3598, 5.9714)
  line L2445 (-131.3598, 5.9714) -> (-130.3757, 8.9224)
  line L2446 (-130.3757, 8.9224) -> (-129.64, 11.9246)
  line L2447 (-129.64, 11.9246) -> (-129.3754, 12.0569)
  line L2448 (-129.3754, 12.0569) -> (-129.1108, 11.9246)
  line L2449 (-129.1108, 11.9246) -> (-127.7175, 10.2672)
  line L2450 (-127.7175, 10.2672) -> (-126.2004, 8.7496)
  line L2451 (-126.2004, 8.7496) -> (-125.3904, 8.6775)
  line L2452 (-125.3904, 8.6775) -> (-124.7452, 9.1464)
  line L2453 (-124.7452, 9.1464) -> (-124.6722, 10.0633)
  line L2454 (-124.6722, 10.0633) -> (-124.4273, 10.898)
  line L2455 (-124.4273, 10.898) -> (-124.0107, 11.6508)
  line L2456 (-124.0107, 11.6508) -> (-123.4223, 12.3214)
  line L2457 (-123.4223, 12.3214) -> (-122.4992, 11.6625)
  line L2458 (-122.4992, 11.6625) -> (-121.7025, 10.8662)
  line L2459 (-121.7025, 10.8662) -> (-122.364, 9.1464)
  line L2460 (-122.364, 9.1464) -> (-123.7389, 6.5591)
  line L2461 (-123.7389, 6.5591) -> (-124.8775, 3.8548)
  line L2462 (-124.8775, 3.8548) -> (-124.1168, 3.1392)
  line L2463 (-124.1168, 3.1392) -> (-123.6207, 2.3274)
  line L2464 (-123.6207, 2.3274) -> (-123.3892, 1.4194)
  line L2465 (-123.3892, 1.4194) -> (-123.4223, 0.4152)
  line L2466 (-123.4223, 0.4152) -> (-122.8389, -0.0511)
  line L2467 (-122.8389, -0.0511) -> (-122.4019, -0.6034)
  line L2468 (-122.4019, -0.6034) -> (-122.1113, -1.2417)
  line L2469 (-122.1113, -1.2417) -> (-121.9671, -1.966)
  line L2470 (-121.9671, -1.966) -> (-126.9942, -1.966)
  line L2471 (-126.9942, -1.966) -> (-126.9338, -1.1835)
  line L2472 (-126.9338, -1.1835) -> (-126.6711, -0.5258)
  line L2473 (-126.6711, -0.5258) -> (-126.2062, 0.0071)
  line L2474 (-126.2062, 0.0071) -> (-125.539, 0.4152)
  line L2475 (-125.539, 0.4152) -> (-125.6887, 1.0986)
  line L2476 (-125.6887, 1.0986) -> (-126.0032, 1.6791)
  line L2477 (-126.0032, 1.6791) -> (-126.4825, 2.1569)
  line L2478 (-126.4825, 2.1569) -> (-127.1265, 2.5319)
  line L2479 (-127.1265, 2.5319) -> (-127.9729, 2.3096)
  line L2480 (-127.9729, 2.3096) -> (-128.8463, 2.2673)
  line L2481 (-128.8463, 2.2673) -> (-128.5304, 0.1311)
  line L2482 (-128.5304, 0.1311) -> (-128.0525, -1.966)
  line L2483 (-128.0525, -1.966) -> (-138.1067, -1.966)
  line L2484 (-138.1067, -1.966) -> (-138.1067, 2.2673)
  line L2485 (-138.1067, 2.2673) -> (-137.3778, 2.9056)
  line L2486 (-137.3778, 2.9056) -> (-137.1349, 3.5593)
  line L2487 (-137.1349, 3.5593) -> (-137.3778, 4.2285)
  line L2488 (-137.3778, 4.2285) -> (-138.1067, 4.9131)
  line L2489 (-138.1067, 4.9131) -> (-138.1067, 8.0881)
  line L2490 (-138.1067, 8.0881) -> (-136.3974, 8.9662)
  line L2491 (-136.3974, 8.9662) -> (-134.9317, 10.2048)
  line L2492 (-134.9317, 10.2048) -> (-136.4181, 10.9747)
  line L2493 (-136.4181, 10.9747) -> (-138.1067, 11.2631)
  line L2494 (-138.1067, 11.2631) -> (-138.1067, 17.6131)
  line L2495 (-138.1067, 17.6131) -> (-137.3129, 17.6131)
  line L2496 (-137.3129, 17.6131) -> (-137.285, 18.1956)
  line L2497 (-137.285, 18.1956) -> (-137.408, 18.6985)
  line L2498 (-137.408, 18.6985) -> (-137.6819, 19.1217)
  line L2499 (-137.6819, 19.1217) -> (-138.1067, 19.4652)
  line L2500 (-138.1067, 19.4652) -> (-138.1067, 21.8464)
  line L2501 (3.9744, 21.8464) -> (4.3046, 21.7532)
  line L2502 (4.3046, 21.7532) -> (4.5036, 21.4496)
  line L2503 (4.5036, 21.4496) -> (4.2583, 20.7175)
  line L2504 (4.2583, 20.7175) -> (4.5036, 19.9943)
  line L2505 (4.5036, 19.9943) -> (4.1728, 19.399)
  line L2506 (4.1728, 19.399) -> (3.8421, 19.2006)
  line L2507 (3.8421, 19.2006) -> (3.5114, 19.399)
  line L2508 (3.5114, 19.399) -> (3.1807, 19.9943)
  line L2509 (3.1807, 19.9943) -> (3.9744, 21.8464)
  line L2510 (-42.5922, -1.966) -> (-51.588, -1.966)
  line L2511 (-51.588, -1.966) -> (-51.3882, -0.1189)
  line L2512 (-51.3882, -0.1189) -> (-51.4557, 1.7381)
  line L2513 (-51.4557, 1.7381) -> (-51.1727, 2.1062)
  line L2514 (-51.1727, 2.1062) -> (-50.8799, 2.2289)
  line L2515 (-50.8799, 2.2289) -> (-50.5773, 2.1062)
  line L2516 (-50.5773, 2.1062) -> (-50.2651, 1.7381)
  line L2517 (-50.2651, 1.7381) -> (-50.3295, 2.8687)
  line L2518 (-50.3295, 2.8687) -> (-50.7943, 3.9871)
  line L2519 (-50.7943, 3.9871) -> (-53.3078, 4.6485)
  line L2520 (-53.3078, 4.6485) -> (-53.9693, 3.8548)
  line L2521 (-53.9693, 3.8548) -> (-52.9109, -0.2463)
  line L2522 (-52.9109, -0.2463) -> (-53.1755, -1.966)
  line L2523 (-53.1755, -1.966) -> (-61.3776, -1.966)
  line L2524 (-61.3776, -1.966) -> (-61.3776, 2.0027)
  line L2525 (-61.3776, 2.0027) -> (-63.2297, 1.7381)
  line L2526 (-63.2297, 1.7381) -> (-62.6567, 3.9438)
  line L2527 (-62.6567, 3.9438) -> (-61.9068, 6.1037)
  line L2528 (-61.9068, 6.1037) -> (-62.2318, 7.1909)
  line L2529 (-62.2318, 7.1909) -> (-62.7005, 8.2204)
  line L2530 (-62.7005, 8.2204) -> (-62.5682, 9.1464)
  line L2531 (-62.5682, 9.1464) -> (-61.5561, 9.2322)
  line L2532 (-61.5561, 9.2322) -> (-60.7778, 9.6135)
  line L2533 (-60.7778, 9.6135) -> (-60.2332, 10.2905)
  line L2534 (-60.2332, 10.2905) -> (-59.9224, 11.2631)
  line L2535 (-59.9224, 11.2631) -> (-59.4902, 11.4953)
  line L2536 (-59.4902, 11.4953) -> (-58.9963, 11.5277)
  line L2537 (-58.9963, 11.5277) -> (-59.7601, 14.1231)
  line L2538 (-59.7601, 14.1231) -> (-60.187, 16.8194)
  line L2539 (-60.187, 16.8194) -> (-61.3776, 17.6131)
  line L2540 (-61.3776, 17.6131) -> (-61.5149, 18.9486)
  line L2541 (-61.5149, 18.9486) -> (-61.3776, 20.2589)
  line L2542 (-61.3776, 20.2589) -> (-60.9904, 20.4558)
  line L2543 (-60.9904, 20.4558) -> (-60.5838, 20.3912)
  line L2544 (-60.5838, 20.3912) -> (-59.2517, 19.0586)
  line L2545 (-59.2517, 19.0586) -> (-57.8057, 17.8777)
  line L2546 (-57.8057, 17.8777) -> (-57.2766, 18.1423)
  line L2547 (-57.2766, 18.1423) -> (-56.0859, 20.7881)
  line L2548 (-56.0859, 20.7881) -> (-55.767, 21.0284)
  line L2549 (-55.767, 21.0284) -> (-55.4245, 20.7881)
  line L2550 (-55.4245, 20.7881) -> (-55.0552, 19.9474)
  line L2551 (-55.0552, 19.9474) -> (-55.2922, 19.0683)
  line L2552 (-55.2922, 19.0683) -> (-54.3038, 16.6946)
  line L2553 (-54.3038, 16.6946) -> (-53.0432, 14.4381)
  line L2554 (-53.0432, 14.4381) -> (-52.7786, 12.586)
  line L2555 (-52.7786, 12.586) -> (-51.8635, 11.9292)
  line L2556 (-51.8635, 11.9292) -> (-51.0589, 11.1308)
  line L2557 (-51.0589, 11.1308) -> (-50.5297, 10.9985)
  line L2558 (-50.5297, 10.9985) -> (-50.0005, 11.1308)
  line L2559 (-50.0005, 11.1308) -> (-48.6776, 13.6444)
  line L2560 (-48.6776, 13.6444) -> (-47.8531, 12.2631)
  line L2561 (-47.8531, 12.2631) -> (-47.487, 10.7339)
  line L2562 (-47.487, 10.7339) -> (-48.5453, 8.8819)
  line L2563 (-48.5453, 8.8819) -> (-48.683, 6.9827)
  line L2564 (-48.683, 6.9827) -> (-48.5745, 5.1149)
  line L2565 (-48.5745, 5.1149) -> (-48.2199, 3.2785)
  line L2566 (-48.2199, 3.2785) -> (-47.6193, 1.4735)
  line L2567 (-47.6193, 1.4735) -> (-47.8342, 0.5393)
  line L2568 (-47.8342, 0.5393) -> (-47.6193, -0.3785)
  line L2569 (-47.6193, -0.3785) -> (-46.6657, -0.0685)
  line L2570 (-46.6657, -0.0685) -> (-45.8187, 0.3876)
  line L2571 (-45.8187, 0.3876) -> (-45.0782, 0.9898)
  line L2572 (-45.0782, 0.9898) -> (-44.4443, 1.7381)
  line L2573 (-44.4443, 1.7381) -> (-43.411, -0.0639)
  line L2574 (-43.411, -0.0639) -> (-42.5922, -1.966)
  line L2575 (-138.1067, 19.4652) -> (-137.6819, 19.1217)
  line L2576 (-137.6819, 19.1217) -> (-137.408, 18.6985)
  line L2577 (-137.408, 18.6985) -> (-137.285, 18.1956)
  line L2578 (-137.285, 18.1956) -> (-137.3129, 17.6131)
  line L2579 (-137.3129, 17.6131) -> (-138.1067, 17.6131)
  line L2580 (-138.1067, 17.6131) -> (-138.1067, 19.4652)
  line L2581 (1.064, 19.2006) -> (1.5529, 19.0837)
  line L2582 (1.5529, 19.0837) -> (1.7599, 18.9125)
  line L2583 (1.7599, 18.9125) -> (1.6852, 18.6868)
  line L2584 (1.6852, 18.6868) -> (1.3286, 18.4068)
  line L2585 (1.3286, 18.4068) -> (1.0866, 18.769)
  line L2586 (1.0866, 18.769) -> (1.064, 19.2006)
  line L2587 (-61.3776, 17.6131) -> (-61.7745, 14.4381)
  line L2588 (-61.7745, 14.4381) -> (-62.1468, 14.0135)
  line L2589 (-62.1468, 14.0135) -> (-62.7005, 13.9089)
  line L2590 (-62.7005, 13.9089) -> (-62.8698, 16.427)
  line L2591 (-62.8698, 16.427) -> (-62.7005, 18.936)
  line L2592 (-62.7005, 18.936) -> (-61.9632, 18.3311)
  line L2593 (-61.9632, 18.3311) -> (-61.3776, 17.6131)
  line L2594 (-86.7776, 18.6714) -> (-85.9838, 18.6714)
  line L2595 (-85.9838, 18.6714) -> (-86.1717, 17.7664)
  line L2596 (-86.1717, 17.7664) -> (-86.7776, 17.0839)
  line L2597 (-86.7776, 17.0839) -> (-87.0145, 17.8809)
  line L2598 (-87.0145, 17.8809) -> (-86.7776, 18.6714)
  line L2599 (-40.7401, 18.1423) -> (-40.3787, 17.8322)
  line L2600 (-40.3787, 17.8322) -> (-40.2802, 17.5084)
  line L2601 (-40.2802, 17.5084) -> (-40.4448, 17.1708)
  line L2602 (-40.4448, 17.1708) -> (-40.8724, 16.8194)
  line L2603 (-40.8724, 16.8194) -> (-40.9663, 17.5004)
  line L2604 (-40.9663, 17.5004) -> (-40.7401, 18.1423)
  line L2605 (-101.065, 17.3485) -> (-100.7021, 17.2994)
  line L2606 (-100.7021, 17.2994) -> (-100.4036, 17.0839)
  line L2607 (-100.4036, 17.0839) -> (-100.3057, 16.0824)
  line L2608 (-100.3057, 16.0824) -> (-100.5359, 15.0996)
  line L2609 (-100.5359, 15.0996) -> (-100.1507, 13.9546)
  line L2610 (-100.1507, 13.9546) -> (-100.0884, 12.8453)
  line L2611 (-100.0884, 12.8453) -> (-100.3491, 11.7718)
  line L2612 (-100.3491, 11.7718) -> (-100.9328, 10.7339)
  line L2613 (-100.9328, 10.7339) -> (-101.6332, 11.8702)
  line L2614 (-101.6332, 11.8702) -> (-102.1234, 13.1152)
  line L2615 (-102.1234, 13.1152) -> (-101.4299, 15.1923)
  line L2616 (-101.4299, 15.1923) -> (-101.065, 17.3485)
  line L2617 (-120.115, 16.8194) -> (-119.3213, 16.8194)
  line L2618 (-119.3213, 16.8194) -> (-119.4689, 16.01)
  line L2619 (-119.4689, 16.01) -> (-120.115, 15.4964)
  line L2620 (-120.115, 15.4964) -> (-120.3465, 16.158)
  line L2621 (-120.3465, 16.158) -> (-120.115, 16.8194)
  line L2622 (-78.3109, -1.966) -> (-82.8088, -1.966)
  line L2623 (-82.8088, -1.966) -> (-82.6765, -0.3785)
  line L2624 (-82.6765, -0.3785) -> (-81.454, 1.6399)
  line L2625 (-81.454, 1.6399) -> (-79.7661, 3.3256)
  line L2626 (-79.7661, 3.3256) -> (-79.3476, 4.6235)
  line L2627 (-79.3476, 4.6235) -> (-79.1047, 5.9714)
  line L2628 (-79.1047, 5.9714) -> (-79.6922, 8.0573)
  line L2629 (-79.6922, 8.0573) -> (-80.0307, 10.2048)
  line L2630 (-80.0307, 10.2048) -> (-81.6355, 12.3423)
  line L2631 (-81.6355, 12.3423) -> (-82.9411, 14.7027)
  line L2632 (-82.9411, 14.7027) -> (-83.0683, 15.5121)
  line L2633 (-83.0683, 15.5121) -> (-82.8088, 16.2902)
  line L2634 (-82.8088, 16.2902) -> (-81.421, 15.6178)
  line L2635 (-81.421, 15.6178) -> (-79.8984, 15.3641)
  line L2636 (-79.8984, 15.3641) -> (-79.1047, 14.0412)
  line L2637 (-79.1047, 14.0412) -> (-78.1786, 13.9089)
  line L2638 (-78.1786, 13.9089) -> (-73.2838, 15.4964)
  line L2639 (-73.2838, 15.4964) -> (-73.3758, 14.8237)
  line L2640 (-73.3758, 14.8237) -> (-73.813, 14.3058)
  line L2641 (-73.813, 14.3058) -> (-75.9132, 13.1238)
  line L2642 (-75.9132, 13.1238) -> (-77.914, 11.7923)
  line L2643 (-77.914, 11.7923) -> (-77.9934, 9.3856)
  line L2644 (-77.9934, 9.3856) -> (-77.5172, 7.0298)
  line L2645 (-77.5172, 7.0298) -> (-78.4432, 5.4423)
  line L2646 (-78.4432, 5.4423) -> (-78.7148, 3.5872)
  line L2647 (-78.7148, 3.5872) -> (-78.7833, 1.7342)
  line L2648 (-78.7833, 1.7342) -> (-78.6487, -0.117)
  line L2649 (-78.6487, -0.117) -> (-78.3109, -1.966)
  line L2650 (0.0057, 15.761) -> (1.3286, 13.7766)
  line L2651 (1.3286, 13.7766) -> (2.8161, 13.2039)
  line L2652 (2.8161, 13.2039) -> (3.8632, 12.2854)
  line L2653 (3.8632, 12.2854) -> (4.4698, 11.0211)
  line L2654 (4.4698, 11.0211) -> (4.6359, 9.411)